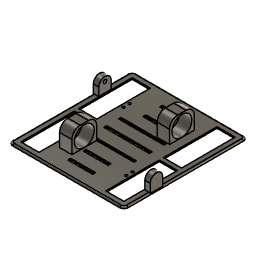
Chassis V3 v4 (Autodesk Fusion 360 design; units mm, degrees)
Autodesk Fusion 360 part; units mm, degrees
sketch "Sketch1" plane through (0, 0, 0) normal (0, 0, 1) x (1, 0, 0)
  line L0 (0, 0) -> (140, 0)
  line L1 (140, 0) -> (140, 150)
  line L2 (140, 150) -> (0, 150)
  line L3 (0, 150) -> (0, 0)
  dimension "d1" = 140
  dimension "d2" = 150
  constraint horizontal L0
  constraint vertical L1
  constraint horizontal L2
  constraint vertical L3
  constraint coincident L0.start L3.end
  measures "d1" distance of L0.start L0.end
  measures "d2" distance of L0.start L2.end
extrude "Extrude1" add sketch "Sketch1" along normal blind 1.75
sketch "Sketch2" plane through (0, 0, 1.75) normal (0, 0, 1) x (-1, 0, 0)
  line L0 (0, -150) -> (0, 0)
  line L1 (0, 0) -> (-140, 0)
  line L2 (-140, 0) -> (-140, -150)
  line L3 (-140, -150) -> (0, -150)
  line L4 (-7.5, -7.5) -> (-132.5, -7.5)
  line L5 (-132.5, -7.5) -> (-132.5, -142.5)
  line L6 (-132.5, -142.5) -> (-7.5, -142.5)
  line L7 (-7.5, -142.5) -> (-7.5, -7.5)
  line L8 (-7.5, -142.5) -> (-29.5, -142.5)
  line L9 (-29.5, -142.5) -> (-29.5, -77.5)
  line L10 (-29.5, -77.5) -> (-7.5, -77.5)
  line L11 (-7.5, -77.5) -> (-7.5, -142.5)
  line L12 (-132.5, -142.5) -> (-132.5, -77.5)
  line L13 (-110.5, -142.5) -> (-132.5, -142.5)
  line L14 (-132.5, -77.5) -> (-110.5, -77.5)
  line L15 (-110.5, -77.5) -> (-110.5, -142.5)
  line L16 (-29.5, -72.5) -> (-29.5, -7.5)
  line L17 (-7.5, -72.5) -> (-29.5, -72.5)
  line L18 (-29.5, -7.5) -> (-7.5, -7.5)
  line L19 (-7.5, -7.5) -> (-7.5, -72.5)
  line L20 (-132.5, -72.5) -> (-132.5, -7.5)
  line L21 (-110.5, -72.5) -> (-132.5, -72.5)
  line L22 (-132.5, -7.5) -> (-110.5, -7.5)
  line L23 (-110.5, -7.5) -> (-110.5, -72.5)
  dimension "d5" = -7.5
  dimension "d6" = 22
  dimension "d7" = 65
  dimension "d10" = -103
  dimension "d11" = 70
  constraint horizontal L8
  constraint vertical L9
  constraint horizontal L10
  constraint vertical L11
  measures "d6" distance of L6.end L8.end
  measures "d7" distance of L6.end L10.end
extrude "Extrude2" cut sketch "Sketch2" against normal up to surface (1.75 mm away) contours L4 L7 L16 L17 L18 L19 | L4 L5 L20 L21 L22 L23 | L6 L7 L8 L9 L10 L11 | L5 L6 L12 L13 L14 L15
sketch "Sketch3" plane through (0, 0, 1.75) normal (0, 0, 1) x (-1, 0, 0)
  line L0 (-110.5, -7.5) -> (-110.5, -72.5)
  line L1 (-132.5, -72.5) -> (-132.5, -7.5)
  line L2 (-132.5, -7.5) -> (-110.5, -7.5)
  line L3 (-110.5, -77.5) -> (-110.5, -142.5)
  line L4 (-110.5, -142.5) -> (-132.5, -142.5)
  line L5 (-132.5, -142.5) -> (-132.5, -77.5)
  line L6 (-132.5, -77.5) -> (-110.5, -77.5)
  line L7 (-7.5, -77.5) -> (-7.5, -142.5)
  line L8 (-7.5, -142.5) -> (-29.5, -142.5)
  line L9 (-29.5, -142.5) -> (-29.5, -77.5)
  line L10 (-29.5, -77.5) -> (-7.5, -77.5)
  line L11 (-7.5, -7.5) -> (-7.5, -72.5)
  line L12 (-29.5, -72.5) -> (-29.5, -7.5)
  line L13 (-29.5, -7.5) -> (-7.5, -7.5)
  line L14 (0, -150) -> (0, 0)
  line L15 (0, 0) -> (-140, 0)
  line L16 (-140, 0) -> (-140, -150)
  line L17 (-140, -150) -> (0, -150)
  line L18 (-29.5, -110) -> (-110.5, -110) construction
  line L19 (-29.5, -40) -> (-110.5, -40) construction
  line L20 (-29.5, -110) -> (-33.25, -110) construction
  line L21 (-30.0705, -117.5) -> (-36.4295, -117.5)
  line L22 (-36.4295, -117.5) -> (-36.4295, -102.5)
  line L23 (-36.4295, -102.5) -> (-30.0705, -102.5)
  line L24 (-30.0705, -102.5) -> (-30.0705, -117.5)
  line L25 (-30.0705, -117.5) -> (-36.4295, -102.5) construction
  line L26 (-36.4295, -117.5) -> (-30.0705, -102.5) construction
  line L27 (-103.5705, -47.5) -> (-109.9295, -47.5)
  line L28 (-103.5705, -32.5) -> (-103.5705, -47.5)
  line L29 (-109.9295, -32.5) -> (-103.5705, -32.5)
  line L30 (-109.9295, -47.5) -> (-109.9295, -32.5)
  line L31 (-110.5, -110) -> (-140, -110) construction
  line L32 (-33.25, -117.5) -> (-33.25, -110) construction
  line L33 (-33.25, -110) -> (-33.25, -102.5) construction
  circle A0 centre (-33.25, -113.75) radius 1.5
  circle A1 centre (-33.25, -106.25) radius 1.5
  line L34 (-106.75, -47.5) -> (-106.75, -40) construction
  line L35 (-106.75, -40) -> (-106.75, -32.5) construction
  circle A2 centre (-106.75, -43.75) radius 1.5
  circle A3 centre (-106.75, -36.25) radius 1.5
  line L36 (-7.5, -110) -> (0, -110) construction
  line L37 (-7.0568, -117.5) -> (-0.4432, -117.5)
  line L38 (-0.4432, -117.5) -> (-0.4432, -102.5)
  line L39 (-0.4432, -102.5) -> (-7.0568, -102.5)
  line L40 (-7.0568, -102.5) -> (-7.0568, -117.5)
  line L41 (-7.0568, -117.5) -> (-0.4432, -102.5) construction
  line L42 (-0.4432, -117.5) -> (-7.0568, -102.5) construction
  line L43 (-139.5568, -47.5) -> (-132.9432, -47.5)
  line L44 (-139.5568, -32.5) -> (-139.5568, -47.5)
  line L45 (-132.9432, -32.5) -> (-139.5568, -32.5)
  line L46 (-132.9432, -47.5) -> (-132.9432, -32.5)
  line L47 (-110.5, -72.5) -> (-132.5, -72.5)
  line L48 (-7.5, -72.5) -> (-29.5, -72.5)
  point P0 (-33.25, -110)
  point P1 (-3.75, -110)
  dimension "d14" = 3.75
  dimension "d15" = 15
  dimension "d18" = -73.5
  dimension "d19" = 70
  dimension "d26" = 3
  dimension "d27" = 3
  dimension "d28" = 3
  dimension "d29" = 3
  dimension "d49" = 15
  dimension "d52" = -132.5
  dimension "d53" = 70
  constraint midpoint L9 L18.start
  constraint midpoint L3 L18.end
  constraint midpoint L12 L19.start
  constraint midpoint L0 L19.end
  constraint perpendicular L9 L20
  constraint horizontal L21
  constraint perpendicular L21 L22
  constraint parallel L21 L23
  constraint parallel L22 L24
  constraint coincident L25 P0
  constraint coincident L26 P0
  constraint coincident P0 L20.end
  constraint coincident L16 L31.end
  constraint perpendicular L16 L31
  constraint midpoint L21 L32.start
  constraint midpoint L23 L33.end
  constraint midpoint L32 A0.centre
  constraint midpoint L33 A1.centre
  constraint midpoint L27 L34.start
  constraint coincident L19 L34.end
  constraint perpendicular L19 L34
  constraint midpoint L29 L35.end
  constraint midpoint L34 A2.centre
  constraint midpoint L35 A3.centre
  constraint midpoint L7 L36.start
  constraint coincident L14 L36.end
  constraint perpendicular L14 L36
  constraint horizontal L37
  constraint perpendicular L37 L38
  constraint parallel L37 L39
  constraint parallel L38 L40
  constraint coincident L41 P1
  constraint coincident L42 P1
  constraint midpoint L36 P1
  measures "d14" distance of L18.start P0
  measures "d15" distance of L21.end L22.end
  measures "d26" diameter of A0
  measures "d27" diameter of A1
  measures "d28" diameter of A2
  measures "d29" diameter of A3
  measures "d49" distance of L37.end L38.end
extrude "Extrude3" add sketch "Sketch3" along normal blind 17.5 contours L37 L38 L39 L40 | L43 L44 L45 L46
extrude "Extrude4" cut sketch "Sketch3" against normal up to surface (1.75 mm away) contours A0 | A1 | A2 | A3
sketch "Sketch4" plane through (132.5, 0, 0) normal (-1, 0, 0) x (0, -1, 0)
  line L0 (-72.5, 0) -> (-7.5, 0)
  line L1 (-7.5, 0) -> (-7.5, 1.75)
  line L2 (-72.5, 1.75) -> (-7.5, 1.75) construction
  line L3 (-40, 1.75) -> (-40, 13.875) construction
  circle A0 centre (-40, 13.875) radius 2.15
  line L4 (-72.5, 1.75) -> (-72.5, 0)
  line L5 (-7.5, 1.75) -> (-72.5, 1.75)
  dimension "d32" = 12.125
  dimension "d33" = 4.3
  constraint midpoint L2 L3.start
  constraint coincident L3.end A0.centre
  measures "d32" distance of L3.start L3.end
  measures "d33" diameter of A0
sketch "Sketch5" plane through (7.5, 0, 0) normal (1, 0, 0) x (0, 1, 0)
  line L0 (77.5, 0) -> (142.5, 0)
  line L1 (142.5, 0) -> (142.5, 1.75)
  line L2 (77.5, 1.75) -> (77.5, 0)
  line L3 (110, 1.75) -> (110, 13.875) construction
  circle A0 centre (110, 13.875) radius 2.15
  line L4 (142.5, 1.75) -> (77.5, 1.75)
  dimension "d34" = 12.125
  dimension "d35" = 4.3
  constraint coincident L3.end A0.centre
  constraint midpoint L3.start L4
  constraint perpendicular L3 L4
  measures "d34" distance of L3.start L3.end
  measures "d35" diameter of A0
extrude "Extrude5" cut sketch "Sketch5" against normal blind 5 contours A0
extrude "Extrude6" cut sketch "Sketch4" against normal blind 5 contours A0
sketch "Sketch6" plane through (0, 0, 1.75) normal (0, 0, 1) x (-1, 0, 0)
  line L0 (-110.4369, -110) -> (-102.9369, -110) construction
  line L1 (-102.9369, -110) -> (-82.9369, -110) construction
  line L2 (-100.4369, -125) -> (-85.4369, -125)
  line L3 (-85.4369, -125) -> (-85.4369, -95)
  line L4 (-85.4369, -95) -> (-100.4369, -95)
  line L5 (-100.4369, -95) -> (-100.4369, -125)
  line L6 (-100.4369, -125) -> (-85.4369, -95) construction
  line L7 (-85.4369, -125) -> (-100.4369, -95) construction
  line L8 (0, 0) -> (-140, 0)
  line L9 (-70, -150) -> (-70, 0) construction
  line L10 (0, -150) -> (0, 0)
  line L11 (-140, 0) -> (-140, -150)
  line L12 (0, -75) -> (-140, -75) construction
  line L13 (-51.9369, -55) -> (-36.9369, -55)
  line L14 (-51.9369, -25) -> (-51.9369, -55)
  line L15 (-36.9369, -25) -> (-51.9369, -25)
  line L16 (-36.9369, -55) -> (-36.9369, -25)
  line L17 (-29.5, -110) -> (-37, -110) construction
  line L18 (-37, -110) -> (-110.4369, -110) construction
  point P0 (-92.9369, -110)
  dimension "d40" = 7.5
  dimension "d41" = 20
  dimension "d42" = 15
  dimension "d43" = 30
  dimension "d46" = 48.5
  dimension "d47" = 70
  dimension "d48" = 7.5
  constraint horizontal L2
  constraint perpendicular L2 L3
  constraint parallel L2 L4
  constraint parallel L3 L5
  constraint coincident L6 P0
  constraint coincident L7 P0
  constraint midpoint L1 P0
  constraint midpoint L8 L9.end
  constraint midpoint L10 L12.start
  constraint midpoint L11 L12.end
  constraint perpendicular L5 L18
  measures "d40" distance of L0.end L0.start
  measures "d41" distance of L0.end L1.end
  measures "d42" distance of L3.end L4.end
  measures "d43" distance of L2.end L3.end
  measures "d48" distance of L17.start L17.end
extrude "Extrude7" add sketch "Sketch6" along normal blind 26
sketch "Sketch7" plane through (51.9369, 0, 0) normal (1, 0, 0) x (0, 1, 0)
  line L0 (25, 1.75) -> (55, 1.75)
  line L1 (55, 1.75) -> (55, 27.75)
  line L2 (55, 27.75) -> (25, 27.75)
  line L3 (25, 27.75) -> (25, 1.75)
  line L4 (40, 1.75) -> (40, 26) construction
  circle A0 centre (40, 13.875) radius 12.125
  dimension "d56" = 24.25
  dimension "d57" = 24.25
  constraint midpoint L0 L4.start
  constraint perpendicular L0 L4
  constraint midpoint L4 A0.centre
  measures "d56" distance of L4.start L4.end
  measures "d57" diameter of A0
sketch "Sketch8" plane through (85.4369, 0, 0) normal (-1, 0, 0) x (0, -1, 0)
  line L0 (-125, 1.75) -> (-95, 1.75)
  line L1 (-95, 1.75) -> (-95, 27.75)
  line L2 (-95, 27.75) -> (-125, 27.75)
  line L3 (-125, 27.75) -> (-125, 1.75)
  line L4 (-110, 1.75) -> (-110, 26) construction
  circle A0 centre (-110, 13.875) radius 12.125
  dimension "d58" = 24.25
  dimension "d59" = 24.25
  constraint midpoint L0 L4.start
  constraint perpendicular L0 L4
  constraint midpoint L4 A0.centre
  measures "d58" distance of L4.start L4.end
  measures "d59" diameter of A0
extrude "Extrude8" cut sketch "Sketch8" against normal up to surface (15 mm away) contours A0
extrude "Extrude9" cut sketch "Sketch7" against normal blind 15 contours A0
fillet "Fillet1" radius 5 4 edges at (0, 0, 0.875) (140, 0, 0.875) (140, 150, 0.875) (0, 150, 0.875)
fillet "Fillet2" radius 2 5 edges at (140, 75, 1.75) (138.5355, 148.5355, 1.75) (70, 150, 1.75) (1.4645, 148.5355, 1.75) (0, 75, 1.75)
fillet "Fillet4" radius 10 4 edges at (92.9369, 95, 27.75) (92.9369, 125, 27.75) (44.4369, 55, 27.75) (44.4369, 25, 27.75)
fillet "Fillet5" radius 7.5 4 edges at (136.25, 47.5, 19.25) (136.25, 32.5, 19.25) (3.75, 102.5, 19.25) (3.75, 117.5, 19.25)
sketch "Sketch9" plane through (0, 0, 0) normal (0, 0, -1) x (1, 0, 0)
  circle A0 centre (33.25, -106.25) radius 1.5
  circle A1 centre (106.75, -43.75) radius 1.5
  circle A2 centre (33.25, -113.75) radius 1.5
  circle A3 centre (106.75, -36.25) radius 1.5
  line L0 (110.5, -142.5) -> (110.5, -77.5)
  line L1 (110.5, -77.5) -> (132.5, -77.5)
  line L2 (132.5, -77.5) -> (132.5, -142.5)
  line L3 (132.5, -142.5) -> (110.5, -142.5)
  line L4 (7.5, -72.5) -> (7.5, -7.5)
  line L5 (7.5, -7.5) -> (29.5, -7.5)
  line L6 (29.5, -7.5) -> (29.5, -72.5)
  line L7 (29.5, -72.5) -> (7.5, -72.5)
  line L8 (110.5, -72.5) -> (110.5, -7.5)
  line L9 (110.5, -7.5) -> (132.5, -7.5)
  line L10 (132.5, -7.5) -> (132.5, -72.5)
  line L11 (132.5, -72.5) -> (110.5, -72.5)
  line L12 (7.5, -142.5) -> (7.5, -77.5)
  line L13 (7.5, -77.5) -> (29.5, -77.5)
  line L14 (29.5, -77.5) -> (29.5, -142.5)
  line L15 (29.5, -142.5) -> (7.5, -142.5)
  arc A4 (0, -145) -> (5, -150) centre (5, -145) ccw
  line L16 (5, -150) -> (135, -150)
  arc A5 (135, -150) -> (140, -145) centre (135, -145) ccw
  line L17 (140, -145) -> (140, -5)
  arc A6 (140, -5) -> (135, 0) centre (135, -5) ccw
  line L18 (135, 0) -> (5, 0)
  arc A7 (5, 0) -> (0, -5) centre (5, -5) ccw
  line L19 (0, -5) -> (0, -145)
  line L20 (70, 0) -> (70, -150) construction
  line L21 (0, -75) -> (140, -75) construction
  line L22 (0, 0) -> (0, -75) construction
  line L23 (0, 0) -> (0, -75) construction
  line L24 (0, -37.5) -> (140, -37.5) construction
  line L25 (0, -75) -> (0, -145) construction
  line L26 (0, -110) -> (140, -110) construction
  line L27 (85, -35.75) -> (55, -35.75)
  line L28 (55, -35.75) -> (55, -39.25)
  line L29 (55, -39.25) -> (85, -39.25)
  line L30 (85, -39.25) -> (85, -35.75)
  line L31 (85, -35.75) -> (55, -39.25) construction
  line L32 (55, -35.75) -> (85, -39.25) construction
  line L33 (97.5, -73.25) -> (42.5, -73.25)
  line L34 (42.5, -73.25) -> (42.5, -76.75)
  line L35 (42.5, -76.75) -> (97.5, -76.75)
  line L36 (97.5, -76.75) -> (97.5, -73.25)
  line L37 (97.5, -73.25) -> (42.5, -76.75) construction
  line L38 (42.5, -73.25) -> (97.5, -76.75) construction
  line L39 (85, -108.25) -> (55, -108.25)
  line L40 (55, -108.25) -> (55, -111.75)
  line L41 (55, -111.75) -> (85, -111.75)
  line L42 (85, -111.75) -> (85, -108.25)
  line L43 (85, -108.25) -> (55, -111.75) construction
  line L44 (55, -108.25) -> (85, -111.75) construction
  line L45 (0, 0) -> (0, -37.5) construction
  line L46 (0, -37.5) -> (0, -75) construction
  line L47 (0, -75) -> (0, -110) construction
  line L48 (0, -110) -> (0, -150.5) construction
  line L49 (0, -18.75) -> (140, -18.75) construction
  line L50 (0, -56.25) -> (140, -56.25) construction
  line L51 (0, -92.5) -> (140, -92.5) construction
  line L52 (0, -130.25) -> (140, -130.25) construction
  line L53 (97.5, -54.875) -> (42.5, -54.875)
  line L54 (42.5, -54.875) -> (42.5, -57.625)
  line L55 (42.5, -57.625) -> (97.5, -57.625)
  line L56 (97.5, -57.625) -> (97.5, -54.875)
  line L57 (97.5, -54.875) -> (42.5, -57.625) construction
  line L58 (42.5, -54.875) -> (97.5, -57.625) construction
  line L59 (97.5, -91) -> (42.5, -91)
  line L60 (42.5, -91) -> (42.5, -94)
  line L61 (42.5, -94) -> (97.5, -94)
  line L62 (97.5, -94) -> (97.5, -91)
  line L63 (97.5, -91) -> (42.5, -94) construction
  line L64 (42.5, -91) -> (97.5, -94) construction
  line L65 (85, -128.5) -> (55, -128.5)
  line L66 (55, -128.5) -> (55, -132)
  line L67 (55, -132) -> (85, -132)
  line L68 (85, -132) -> (85, -128.5)
  line L69 (85, -128.5) -> (55, -132) construction
  line L70 (55, -128.5) -> (85, -132) construction
  line L71 (85, -17) -> (55, -17)
  line L72 (55, -17) -> (55, -20.5)
  line L73 (55, -20.5) -> (85, -20.5)
  line L74 (85, -20.5) -> (85, -17)
  line L75 (85, -17) -> (55, -20.5) construction
  line L76 (55, -17) -> (85, -20.5) construction
  point P0 (70, -37.5)
  point P1 (70, -75)
  point P2 (70, -110)
  point P3 (70, -56.25)
  point P4 (70, -92.5)
  point P5 (70, -130.25)
  point P6 (70, -18.75)
  dimension "d74" = 30
  dimension "d75" = 3.5
  dimension "d76" = 55
  dimension "d77" = 3.5
  dimension "d78" = 30
  dimension "d79" = 3.5
  dimension "d82" = 55
  dimension "d83" = 2.75
  dimension "d84" = 55
  dimension "d85" = 3
  dimension "d86" = 30
  dimension "d87" = 3.5
  dimension "d88" = 30
  dimension "d89" = 3.5
  constraint midpoint L18 L20.start
  constraint midpoint L16 L20.end
  constraint midpoint L19 L21.start
  constraint midpoint L17 L21.end
  constraint coincident L22.start L23.start
  constraint midpoint L23 L24.start
  constraint coincident L17 L24.end
  constraint perpendicular L17 L24
  constraint perpendicular L16 L25
  constraint midpoint L25 L26.start
  constraint coincident L17 L26.end
  constraint perpendicular L17 L26
  constraint horizontal L27
  constraint perpendicular L27 L28
  constraint parallel L27 L29
  constraint parallel L28 L30
  constraint coincident L31 P0
  constraint coincident L32 P0
  constraint midpoint L24 P0
  constraint horizontal L33
  constraint perpendicular L33 L34
  constraint parallel L33 L35
  constraint parallel L34 L36
  constraint coincident L37 P1
  constraint coincident L38 P1
  constraint midpoint L20 P1
  constraint horizontal L39
  constraint perpendicular L39 L40
  constraint parallel L39 L41
  constraint parallel L40 L42
  constraint coincident L43 P2
  constraint coincident L44 P2
  constraint midpoint L26 P2
  constraint perpendicular L16 L48
  constraint midpoint L45 L49.start
  constraint coincident L17 L49.end
  constraint perpendicular L17 L49
  constraint midpoint L46 L50.start
  constraint coincident L17 L50.end
  constraint perpendicular L17 L50
  constraint midpoint L47 L51.start
  constraint coincident L17 L51.end
  constraint perpendicular L17 L51
  constraint midpoint L48 L52.start
  constraint coincident L17 L52.end
  constraint perpendicular L17 L52
  constraint horizontal L53
  constraint perpendicular L53 L54
  constraint parallel L53 L55
  constraint parallel L54 L56
  constraint coincident L57 P3
  constraint coincident L58 P3
  constraint midpoint L50 P3
  constraint horizontal L59
  constraint perpendicular L59 L60
  constraint parallel L59 L61
  constraint parallel L60 L62
  constraint coincident L63 P4
  constraint coincident L64 P4
  constraint midpoint L51 P4
  constraint horizontal L65
  constraint perpendicular L65 L66
  constraint parallel L65 L67
  constraint parallel L66 L68
  constraint coincident L69 P5
  constraint coincident L70 P5
  constraint midpoint L52 P5
  constraint horizontal L71
  constraint perpendicular L71 L72
  constraint parallel L71 L73
  constraint parallel L72 L74
  constraint coincident L75 P6
  constraint coincident L76 P6
  constraint midpoint L49 P6
  measures "d74" distance of L28.end L29.end
  measures "d75" distance of L27.end L28.end
  measures "d76" distance of L34.end L35.end
  measures "d77" distance of L33.end L34.end
  measures "d78" distance of L40.end L41.end
  measures "d79" distance of L39.end L40.end
  measures "d82" distance of L54.end L55.end
  measures "d83" distance of L53.end L54.end
  measures "d84" distance of L60.end L61.end
  measures "d85" distance of L59.end L60.end
  measures "d86" distance of L66.end L67.end
  measures "d87" distance of L65.end L66.end
  measures "d88" distance of L72.end L73.end
  measures "d89" distance of L71.end L72.end
extrude "Extrude10" cut sketch "Sketch9" against normal up to surface (1.75 mm away) contours L27 L28 L29 L30 | L33 L34 L35 L36 | L39 L40 L41 L42 | L53 L54 L55 L56 | L59 L60 L61 L62 | L65 L66 L67 L68 | L71 L72 L73 L74
